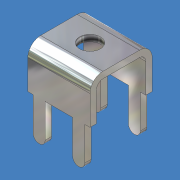
# Autodesk Inventor part: BreakerPanelScrewTerminal
Saved by Autodesk Inventor 2011 SP1 (Build 150282100, 282)
## iProperties
Shininess: 86.0
Length Units: 11272
Angle Units: 11279
Time Units: 11290
Mass Units: 11286
Length Display Precision: 3
Angle Display Precision: 2
Created: 2005-12-06
Part Number: BreakerPanelScrewTerminal
Material: Bronze, Soft Tin
Document SubType Name: Sheet Metal
Designer: t8558es
Density: 1 g/cm^3
Sheet Metal Rule: Default
Density: 0.0
Volumn: 0.0
Area: 0.0
PropertySet Name: Model Information
Control State: 0
Master: False
Checked Out: False
Author: t8558es
Autodesk Inventor part; units mm, degrees
ref_plane "YZ Plane" through (0, 0, 0) normal (1, 0, 0) x (0, 1, 0)
ref_plane "XZ Plane" through (0, 0, 0) normal (0, 1, 0) x (-1, 0, 0)
ref_plane "XY Plane" through (0, 0, 0) normal (0, 0, 1) x (1, 0, 0)
sketch "Sketch1" plane through (0, 0, 0) normal (0, 0, 1) x (1, 0, 0)
  line L0 (0, 7.874) -> (7.874, 7.874)
  line L1 (7.874, 7.874) -> (7.874, 0)
  line L2 (7.874, 0) -> (0, 0)
  line L3 (0, 0) -> (0, 7.874)
  dimension "d0" = 7.874
  dimension "d1" = 7.874
  measures "d0" distance of L0.start L0.end
  measures "d1" distance of L0.end L1.end
extrude "Plate1" add sketch "Sketch1" along normal blind 0.8128
sketch "Sketch2" plane through (7.874, 7.874, 0) normal (0, -1, 0) x (-1, 0, 0)
  line L0 (0, 0) -> (7.874, 0)
  line L1 (7.874, 0) -> (7.874, -5.334)
  line L2 (7.874, -5.334) -> (0, -5.334)
  line L3 (0, -5.334) -> (0, 0)
  constraints: 4 end point, 4 other
sheet face with bend "Flange1" sketch "Sketch2" thickness 0.8128 toward (0, -1, 0) bend radius 0.8128 relief straight relief width 0.8128 relief depth 0.4064
bend "Bend1"
sketch "Sketch3" plane through (0, 0, 0) normal (0, 1, 0) x (1, 0, 0)
  line L0 (0, 0) -> (7.874, 0)
  line L1 (7.874, 0) -> (7.874, -5.334)
  line L2 (7.874, -5.334) -> (0, -5.334)
  line L3 (0, -5.334) -> (0, 0)
  constraints: 4 end point, 4 other
sheet face with bend "Flange2" sketch "Sketch3" thickness 0.8128 toward (0, 1, 0) bend radius 0.8128 relief straight relief width 0.8128 relief depth 0.4064
bend "Bend2"
sketch "Sketch4" plane through (7.874, 6.2484, 0) normal (0, 0, -1) x (-1, 0, 0)
  line L0 (0, -4.6228) -> (7.874, -4.6228) projected
  line L1 (7.874, -4.6228) -> (7.874, 0) projected
  line L2 (7.874, 0) -> (0, 0) projected
  line L3 (0, 0) -> (0, -4.6228) projected
  line L4 (3.937, -2.3114) -> (0, -2.3114)
  line L5 (3.937, -2.3114) -> (7.874, -2.3114)
  line L6 (3.937, -2.3114) -> (3.937, 0)
  line L7 (3.937, -2.3114) -> (3.937, -4.6228)
  constraints: 8 end point, 4 midpoint, 3 collinear, 3 perpendicular
hole "Hole1" at (3.937, 3.937, 0) direction (0, 0, 1) diameter 2.6416 end through all thread size "6-32 UNC" class "2B" standard "ANSI Unified Screw Threads"
sketch "Sketch5" plane through (0, 7.0612, 5.334) normal (0, -1, 0) x (1, 0, 0)
  line L0 (0.6731, 0) -> (2.1971, 0)
  line L1 (2.1971, 0) -> (2.1971, 5.0038)
  line L2 (2.1971, 5.0038) -> (0.6731, 5.0038)
  line L3 (0.6731, 5.0038) -> (0.6731, 0)
  constraints: 8 end point
sheet face with bend "Flange3" sketch "Sketch5" thickness 0.8128 toward (0, 1, 0) bend radius 0.8128 relief straight relief width 0.8128 relief depth 0.4064
bend "Bend3"
sketch "Sketch6" plane through (7.874, 7.874, 5.334) normal (0, 1, 0) x (-1, 0, 0)
  line L0 (0.6731, 0) -> (2.1971, 0)
  line L1 (2.1971, 0) -> (2.1971, 5.0038)
  line L2 (2.1971, 5.0038) -> (0.6731, 5.0038)
  line L3 (0.6731, 5.0038) -> (0.6731, 0)
  constraints: 8 end point
sheet face with bend "Flange4" sketch "Sketch6" thickness 0.8128 toward (0, -1, 0) bend radius 0.8128 relief straight relief width 0.8128 relief depth 0.4064
bend "Bend4"
sketch "Sketch7" plane through (0, 0, 5.334) normal (0, -1, 0) x (1, 0, 0)
  line L0 (7.2009, 0) -> (5.6769, 0)
  line L1 (5.6769, 0) -> (5.6769, 5.0038)
  line L2 (5.6769, 5.0038) -> (7.2009, 5.0038)
  line L3 (7.2009, 5.0038) -> (7.2009, 0)
  constraints: 8 end point
sheet face with bend "Flange5" sketch "Sketch7" thickness 0.8128 toward (0, 1, 0) bend radius 0.8128 relief straight relief width 0.8128 relief depth 0.4064
bend "Bend5"
sketch "Sketch8" plane through (0, 0, 5.334) normal (0, -1, 0) x (1, 0, 0)
  line L0 (0.6731, 0) -> (2.1971, 0)
  line L1 (2.1971, 0) -> (2.1971, 5.0038)
  line L2 (2.1971, 5.0038) -> (0.6731, 5.0038)
  line L3 (0.6731, 5.0038) -> (0.6731, 0)
  constraints: 8 end point
sheet face with bend "Flange6" sketch "Sketch8" thickness 0.8128 toward (0, 1, 0) bend radius 0.8128 relief straight relief width 0.8128 relief depth 0.4064
bend "Bend6"
fillet "Corner Round1" radius 0.762 8 edges at (2.1971, 7.4676, 10.3378) (0.6731, 7.4676, 10.3378) (5.6769, 7.4676, 10.3378) (7.2009, 7.4676, 10.3378) (0.6731, 0.4064, 10.3378) (2.1971, 0.4064, 10.3378) (5.6769, 0.4064, 10.3378) (7.2009, 0.4064, 10.3378)
equation "\"d6\" = BendRadius"
equation "\"MinimumRemnant\" = 2 * Thickness"
equation "\"BendReliefWidth\" = Thickness"
equation "\"d3\" = BendRadius"
equation "\"d44\" = BendReliefWidth"
equation "\"d45\" = BendReliefDepth"
equation "\"d46\" = MinimumRemnant"
equation "\"d10\" = BendRadius"
equation "\"d7\" = BendRadius"
equation "\"d47\" = BendReliefWidth"
equation "\"d48\" = BendReliefDepth"
equation "\"d49\" = MinimumRemnant"
equation "\"d23\" = BendRadius"
equation "\"d20\" = BendRadius"
equation "\"d50\" = BendReliefWidth"
equation "\"d51\" = BendReliefDepth"
equation "\"d52\" = MinimumRemnant"
equation "\"d30\" = BendRadius"
equation "\"d27\" = BendRadius"
equation "\"d53\" = BendReliefWidth"
equation "\"d54\" = BendReliefDepth"
equation "\"d55\" = MinimumRemnant"
equation "\"d36\" = BendRadius"
equation "\"d33\" = BendRadius"
equation "\"d56\" = BendReliefWidth"
equation "\"d57\" = BendReliefDepth"
equation "\"d58\" = MinimumRemnant"
equation "\"d42\" = BendRadius"
equation "\"d39\" = BendRadius"
equation "\"d59\" = BendReliefWidth"
equation "\"d60\" = BendReliefDepth"
equation "\"d61\" = MinimumRemnant"
equation "\"BendRadius\" = Thickness"
equation "\"BendReliefDepth\" = 0.5 * Thickness"
equation "\"CornerReliefSize\" = 4 * Thickness"
equation "\"TransitionRadius\" = BendRadius"
equation "\"d2\" = BendRadius"
equation "\"JacobiRadiusSize\" = Thickness"
equation "\"GapSize\" = Thickness"
equation "\"Thickness\" = 0.8128"
body "Solid1"
